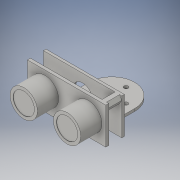
# Autodesk Inventor part: Ultrasound
Saved by Autodesk Inventor 2016 (Build 200138000, 138)
## iProperties
Created: 2015-09-09
Part Number: Ultrasound
Material: Generic
Document SubType Name: Modeling
Designer: lachesis
Density: 1 g/cm^3
Appearance: Default
Author: lachesis
Autodesk Inventor part; units mm, degrees
ref_plane "YZ Plane" through (0, 0, 0) normal (1, 0, 0) x (0, 1, 0)
ref_plane "XZ Plane" through (0, 0, 0) normal (0, 1, 0) x (-1, 0, 0)
ref_plane "XY Plane" through (0, 0, 0) normal (0, 0, 1) x (1, 0, 0)
sketch "Sketch1" plane through (0, 0, 0) normal (0, 0, 1) x (1, 0, 0)
  line L0 (-22.987, 10.668) -> (22.987, 10.668)
  line L1 (22.987, 10.668) -> (22.987, -10.668)
  line L2 (22.987, -10.668) -> (-22.987, -10.668)
  line L3 (-22.987, -10.668) -> (-22.987, 10.668)
  point P0 (0, 0)
  point P1 (-22.987, 0)
  point P2 (0, 10.668)
  dimension "d0" = 45.974
  dimension "d1" = 21.336
  constraints: 8 end point, 2 midpoint, 2 parallel, 1 horizontal, 1 horizontal alignment, 1 perpendicular, 1 vertical alignment
  measures "d0" distance of L0.start L0.end
  measures "d1" distance of L2.end L0.start
extrude "Extrusion1" add sketch "Sketch1" along normal blind 1.778
sketch "Sketch2" plane through (0, 0, 1.778) normal (0, 0, 1) x (1, 0, 0)
  circle A0 centre (-12.7, 0) radius 8.0137
  circle A1 centre (12.7, 0) radius 8.0137
  point P0 (0, 0)
  dimension "d4" = 16.0274
  dimension "d5" = 16.0274
  dimension "d6" = 12.7
  dimension "d7" = 12.7
  constraints: 2 centre point, 2 horizontal alignment
  measures "d4" diameter of A0
  measures "d5" diameter of A1
  measures "d6" distance of A0.centre point (0, 0)
  measures "d7" distance of A1.centre point (0, 0)
extrude "Extrusion2" add sketch "Sketch2" along normal blind 12.4206
sketch "Sketch3" plane through (-12.7, 0, 14.1986) normal (0, 0, 1) x (1, 0, 0)
  circle A0 centre (0, 0) radius 8.0137 projected
  circle A1 centre (25.4, 0) radius 8.0137 projected
  circle A2 centre (0, 0) radius 6.2357
  circle A3 centre (25.4, 0) radius 6.2357
  point P0 (12.7, 0)
  dimension "d11" = 1.778
  dimension "d12" = 1.778
  constraints: 2 centre point, 2 coincident
  measures "d11" radial gap between concentric circles of A2 A0
  measures "d12" radial gap between concentric circles of A1 A3
extrude "Extrusion3" cut sketch "Sketch3" against normal blind 0.254 contours A2 | A3
sketch "Sketch4" plane through (0, 0, 0) normal (0, 0, -1) x (-1, 0, 0)
  line L0 (-19.0275, 6.096) -> (-21.6672, 6.096)
  line L1 (-21.6672, 6.096) -> (-22.987, 8.382)
  line L2 (-22.987, 8.382) -> (-21.6672, 10.668)
  line L3 (-21.6672, 10.668) -> (-19.0275, 10.668)
  line L4 (-19.0275, 10.668) -> (-17.7077, 8.382)
  line L5 (-17.7077, 8.382) -> (-19.0275, 6.096)
  line L6 (21.6672, -10.668) -> (19.0275, -10.668)
  line L7 (19.0275, -10.668) -> (17.7077, -8.382)
  line L8 (17.7077, -8.382) -> (19.0275, -6.096)
  line L9 (19.0275, -6.096) -> (21.6672, -6.096)
  line L10 (21.6672, -6.096) -> (22.987, -8.382)
  line L11 (22.987, -8.382) -> (21.6672, -10.668)
  line L12 (22.987, 10.668) -> (-22.987, 10.668) projected
  line L13 (-22.987, -10.668) -> (22.987, -10.668) projected
  line L14 (22.987, -10.668) -> (22.987, 10.668) projected
  line L15 (-22.987, 10.668) -> (-22.987, -10.668) projected
  point P0 (0, 0)
  point P1 (-20.3474, 8.382)
  point P2 (20.3474, -8.382)
  dimension "d15" = 4.572
  dimension "d16" = 4.572
  constraints: 24 end point, 4 collinear, 2 point on line, 26 other
  measures "d15" distance between parallel lines of L6 L9
  measures "d16" distance between parallel lines of L0 L3
extrude "Extrusion4" add sketch "Sketch4" along normal blind 7.62 contours L0 L1 L2 L3 L4 L5 | L7 L8 L9 L10 L11 L6
sketch "Sketch5" plane through (0, 0, -7.62) normal (0, 0, -1) x (-1, 0, 0)
  line L0 (19.0275, -10.668) -> (17.7077, -8.382) projected
  line L1 (17.7077, -8.382) -> (19.0275, -6.096) projected
  line L2 (19.0275, -6.096) -> (21.6672, -6.096) projected
  line L3 (21.6672, -6.096) -> (22.987, -8.382) projected
  line L4 (22.987, -8.382) -> (22.987, 10.668) projected
  line L5 (22.987, 10.668) -> (-19.0275, 10.668) projected
  line L6 (-19.0275, 10.668) -> (-17.7077, 8.382) projected
  line L7 (-17.7077, 8.382) -> (-19.0275, 6.096) projected
  line L8 (-19.0275, 6.096) -> (-21.6672, 6.096) projected
  line L9 (-21.6672, 6.096) -> (-22.987, 8.382) projected
  line L10 (-22.987, 8.382) -> (-22.987, -10.668) projected
  line L11 (-22.987, -10.668) -> (19.0275, -10.668) projected
  line L12 (-21.6672, 10.668) -> (-22.987, 10.668) projected
  line L13 (-22.987, 10.668) -> (-22.987, 8.382) projected
  line L14 (-19.0275, 10.668) -> (-21.6672, 10.668) projected
  line L15 (19.0275, -10.668) -> (21.6672, -10.668) projected
  line L16 (22.987, -10.668) -> (22.987, -8.382) projected
  line L17 (21.6672, -10.668) -> (22.987, -10.668) projected
  line L18 (-21.6672, 6.096) -> (-19.0275, 6.096) projected
  line L19 (-22.987, 8.382) -> (-21.6672, 6.096) projected
  line L20 (-22.987, 10.668) -> (22.987, 10.668) projected
  line L21 (-22.987, 10.668) -> (22.987, 10.668)
  line L22 (22.987, 10.668) -> (22.987, -10.668)
  line L23 (22.987, -10.668) -> (-22.987, -10.668)
  line L24 (-22.987, -10.668) -> (-22.987, 10.668)
  point P0 (0, 0)
  constraints: 8 end point, 2 parallel, 1 horizontal, 1 perpendicular
extrude "Extrusion5" add sketch "Sketch5" along normal blind 1.524
ref_plane "Work Plane1" through (-22.987, -10.668, 1.778) normal (0, -1, 0) x (1, 0, 0)
sketch "Sketch6" plane through (-22.987, -10.668, 1.778) normal (0, -1, 0) x (1, 0, 0)
  line L0 (0, -1.778) -> (0, -9.398) projected
  line L1 (22.987, -10.922) -> (22.987, -26.543) construction
  line L2 (36.322, -10.922) -> (36.322, -26.543)
  line L3 (9.652, -26.543) -> (9.652, -10.922)
  arc A0 (9.652, -26.543) -> (36.322, -26.543) centre (22.987, -26.543) ccw
  line L4 (0, -10.922) -> (45.974, -10.922) projected
  line L5 (36.322, -10.922) -> (9.652, -10.922)
  point P0 (22.987, -1.778)
  point P1 (22.987, -18.7325)
  point P2 (22.987, -39.878)
  dimension "d23" = 9.652
  dimension "d25" = 26.67
  dimension "d26" = 28.956
  dimension "d27" = 0
  dimension "d28" = 0
  constraints: 10 end point, 3 point on circle, 2 parallel, 2 tangent, 1 centre point, 1 collinear, 1 midpoint
  measures "d23" distance between parallel lines of L3 L0
  measures "d25" distance between parallel lines of L3 L2
  measures "d26" distance from line of L4 point (22.987, -39.878)
  measures "d27" distance between parallel lines of L5 L4
  measures "d28" distance from line of L1.start L4
extrude "Extrusion6" add sketch "Sketch6" against normal blind 1.524
fillet "Fillet1" radius 0.9525 1 edges at (0, -9.144, -9.144)
sketch "Sketch7" plane through (0, 0, -9.144) normal (0, 0, -1) x (-1, 0, 0)
  circle A0 centre (0, 0) radius 5.7785
  dimension "d32" = 11.557
  constraints: 1 centre point, 1 coincident
  measures "d32" diameter of A0
extrude "Extrusion7" cut sketch "Sketch7" against normal up to next
sketch "Sketch8" plane through (-22.987, -10.668, 1.778) normal (0, -1, 0) x (1, 0, 0)
  arc A0 (9.652, -26.543) -> (36.322, -26.543) centre (22.987, -26.543) ccw projected
  line L0 (9.652, -26.543) -> (9.652, -10.922) projected
  line L1 (36.322, -10.922) -> (36.322, -26.543) projected
  circle A1 centre (22.987, -26.543) radius 4.0005
  circle A2 centre (22.987, -34.8742) radius 1.2065
  circle A3 centre (31.3182, -26.543) radius 1.2065
  circle A4 centre (14.6558, -26.543) radius 1.2065
  circle A5 centre (22.987, -18.2118) radius 1.2065
  point P0 (22.987, -1.778)
  dimension "d35" = 8.001
  dimension "d36" = 2.413
  dimension "d37" = 2.413
  dimension "d38" = 2.413
  dimension "d39" = 2.413
  dimension "d40" = 8.3312
  dimension "d41" = 8.3312
  dimension "d42" = 8.3312
  dimension "d43" = 8.3312
  constraints: 5 centre point, 2 horizontal alignment, 2 vertical alignment, 1 coincident
  measures "d35" diameter of A1
  measures "d36" diameter of A2
  measures "d37" diameter of A3
  measures "d38" diameter of A4
  measures "d39" diameter of A5
  measures "d40" distance of A1.centre A2.centre
  measures "d41" distance of A1.centre A3.centre
  measures "d42" distance of A5.centre A1.centre
  measures "d43" distance of A1.centre A4.centre
extrude "Extrusion8" cut sketch "Sketch8" against normal through all
equation "\"d5\" = d4"
equation "\"d7\" = d6"
equation "\"d12\" = d11"
equation "\"d16\" = d15"
equation "\"d37\" = d36"
equation "\"d38\" = d36"
equation "\"d39\" = d36"
equation "\"d41\" = d40"
equation "\"d42\" = d40"
equation "\"d43\" = d40"
body "Solid1"
